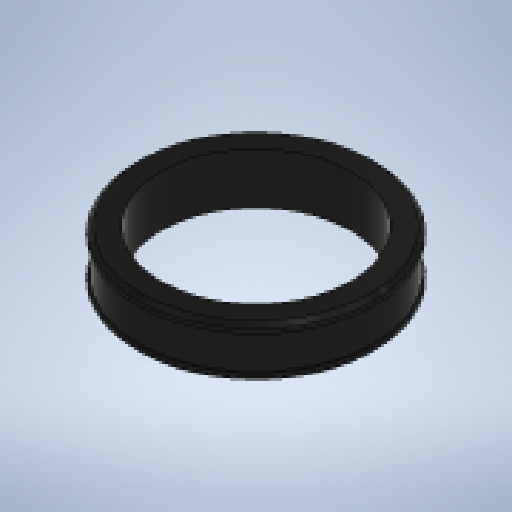
# Autodesk Inventor part: Band - Hub
Saved by Autodesk Inventor 2023.2 (Build 272271000, 271)
## iProperties
Created: 2023-05-10
Part Number: Band - Hub
Material: Nylon 6/6
Document SubType Name: Modeling
Designer: Nathan Cai
Density: 1.13 g/cm^3
Appearance: Smooth - Black
Author: Nathan Cai
Autodesk Inventor part; units mm, degrees
ref_plane "YZ Plane" through (0, 0, 0) normal (1, 0, 0) x (0, 1, 0)
ref_plane "XZ Plane" through (0, 0, 0) normal (0, 1, 0) x (-1, 0, 0)
ref_plane "XY Plane" through (0, 0, 0) normal (0, 0, 1) x (1, 0, 0)
sketch "Sketch1" plane through (0, 0, 0) normal (1, 0, 0) x (0, 1, 0)
  line L0 (0, 0) -> (9.525, 0)
  line L1 (9.525, 0) -> (9.525, -17.675)
  line L2 (9.525, -17.675) -> (0, -17.675)
  line L3 (0, -17.675) -> (0, 0)
  line L4 (0, 0) -> (9.525, 0)
  line L5 (9.525, 0) -> (9.525, -22.225)
  line L6 (9.525, -22.225) -> (0, -22.225)
  line L7 (0, -22.225) -> (0, 0)
  line L8 (1.5875, -21.8281) -> (7.9375, -21.8281)
  line L9 (7.9375, -21.8281) -> (7.9375, -22.6219)
  line L10 (7.9375, -22.6219) -> (1.5875, -22.6219) construction
  line L11 (1.5875, -22.6219) -> (1.5875, -21.8281)
  line L12 (1.5875, -21.8281) -> (7.9375, -22.6219) construction
  line L13 (7.9375, -21.8281) -> (1.5875, -22.6219) construction
  point P0 (4.7625, -22.225)
  point P1 (7.9375, -22.225)
  point P2 (0, -17.675)
  point P3 (1.5875, -22.225)
  dimension "d0" = 17.675
  dimension "d1" = 9.525
  dimension "d2" = 22.225
  dimension "d3" = 6.35
  dimension "d4" = 0.7937
  constraints: 28 end point, 6 parallel, 3 horizontal, 3 midpoint, 3 perpendicular, 1 point on line
  measures "d0" distance of L0.end L1.end
  measures "d1" distance between parallel lines of L3 L1
  measures "d2" distance of L4.end L5.end
  measures "d3" distance of L9.end L10.end
  measures "d4" distance of L8.end L9.end
revolve "Revolution1" add sketch "Sketch1" angle 360 about axis through (0, 0, 0) along (0, 1, 0) contours L2 L5 L6 L9 L8 L11 L7
chamfer "Chamfer1" distance 0.7937 angle 45 2 edges at (0, 9.525, 22.225) (0, 0, 22.225)
body "Solid1"
